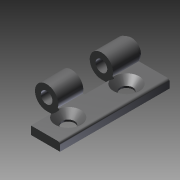
# Autodesk Inventor part: HHPMGS5p2
Saved by Autodesk Inventor 2015 SP1 (Build 190203100, 203)
## iProperties
Category: PARTsolutions
Company: MISUMI
Created: 2015-01-26
Part Number: HHPMGS5p2
Catalog Web Link: www.cadenas.de
Description: HHPMGS_p2-Low Dust Raise Hinges - Part2
Vendor: MISUMI
Document SubType Name: Modeling
Designer: PARTuser1
Manufacturer: MISUMI
Mass: 3.22136 g
Surface Area: 28.5159 cm^2
Volume: 3.22136 cm^3
Density: 1 g/cm^3
Material: Generic
Appearance: PSOLRGB-192-192-192
PSOL_IDENT_0: {\\10.0.0.236\data_v8\23d-libs\misumi\metric\39_accessories_for_al_extrusions\hhpmgs_part2.prj},167
PSOL_IDENT_1: {VTYP=3D},{NB=HHPMGS5p2},{LINA=HHPMGS5p2},{NN=HHPMGS_p2},{DATE=17.11.2014 05:31:03},{GEOMDATE=10.08.
PSOL_IDENT_2: 2009 11:07:00},{VERSION=},{LINEID=10},{LINESUBID=-1},{WBVAR=ALT1}  {NB=HHPMGS5p2},{LINA=HHPMGS5p2},{
PSOL_IDENT_3: KT=DUMMY},{PN=HHPMGS5},{TYPE=HHPMGS},{MAT=6063S-T5 Aluminum Alloy},{MATB=Oil Soaked Polyacetal},{ST=
PSOL_IDENT_4: Electroless Nickel Plating},{NO=5},{ALKG=10},{ALN=98},{MASS=22},{L=47},{W=36},{K=11.0},{P=25},{J=7.5
PSOL_IDENT_5: },{S=21},{ND=5.5},{NC=11},{T=3.5},{E=5.0},{R=5.0},{AB=FB5-8},{ABQ=4},{AN=HNTT5-5},{ANQ=4},{ALT1=},{A
PSOL_IDENT_6: BM=5},{ABL=8},{ANNO=5},{ANM=5}
SUPPLIER: MISUMI
ARTICLENO: HHPMGS5p2
BOMINFO: HHPMGS5p2
CREATOR: CADENAS GmbH
Title: HHPMGS5p2
Author: Cadenas PARTsolutions
Comments: Low Dust Raise Hinges - Part2
Autodesk Inventor part; units mm, degrees
sketch "Sketch_1" plane through (0, 0, 0) normal (0, 1, 0) x (-1, 0, 0)
  arc A0 (0, -5) -> (-4.7697, -1.5) centre (0, 0) ccw
  line L0 (-4.7697, -1.5) -> (-17, -1.5)
  arc A1 (-17, -1.5) -> (-18, -2.5) centre (-17, -2.5) ccw
  line L1 (-18, -2.5) -> (-18, -5)
  line L2 (-18, -5) -> (0, -5)
  circle A2 centre (0, 0) radius 2.5
  constraints: 6 end point, 4 point on circle, 3 centre point
extrude "Extrusion1" add sketch "Sketch_1" along normal mid plane 47
sketch "Sketch_2" plane through (0, 0, 0) normal (0, 0, 1) x (1, 0, 0)
  line L0 (-10, -23.5) -> (5.5, -23.5)
  line L1 (5.5, -23.5) -> (5.5, -11.25)
  line L2 (5.5, -11.25) -> (-5, -11.25)
  line L3 (-5, -11.25) -> (-5, -0.5)
  line L4 (-5, -0.5) -> (5.5, -0.5)
  line L5 (5.5, -0.5) -> (5.5, 12.25)
  line L6 (5.5, 12.25) -> (-5, 12.25)
  line L7 (-5, 12.25) -> (-5, 23.5)
  line L8 (-5, 23.5) -> (-10, 23.5)
  line L9 (-10, 23.5) -> (-10, -23.5)
  constraints: 20 end point
extrude "Extrusion2" cut sketch "Sketch_2" along normal mid plane 10
sketch "Sketch_4" plane through (10.5, 0, 0) normal (1, 0, 0) x (0, 0, -1)
  line L0 (5, 12.5) -> (1.5, 12.5)
  line L1 (1.5, 12.5) -> (1.5, 18)
  line L2 (1.5, 18) -> (4.25, 15.25)
  line L3 (4.25, 15.25) -> (5, 15.25)
  line L4 (5, 15.25) -> (5, 12.5)
  line L5 (5, 12.5) -> (1.5, 12.5)
  constraints: 12 end point
revolve "Revolution1" cut sketch "Sketch_4" angle 360 about axis through (10.5, 12.5, -5) along (0, 0, -1)
sketch "Sketch_5" plane through (10.5, 0, 0) normal (1, 0, 0) x (0, 0, -1)
  line L0 (5, -12.5) -> (1.5, -12.5)
  line L1 (1.5, -12.5) -> (1.5, -7)
  line L2 (1.5, -7) -> (4.25, -9.75)
  line L3 (4.25, -9.75) -> (5, -9.75)
  line L4 (5, -9.75) -> (5, -12.5)
  line L5 (5, -12.5) -> (1.5, -12.5)
  constraints: 12 end point
revolve "Revolution2" cut sketch "Sketch_5" angle 360 about axis through (10.5, -12.5, -5) along (0, 0, -1)
sketch "Sketch_10" plane through (0, 0, 0) normal (0, 0, 1) x (1, 0, 0)
  line L0 (0, 23.5) -> (0, 25.2)
  line L1 (2.5, 23.5) -> (4.5, 23.5)
  line L2 (4.5, 23.5) -> (4.5, 24.5)
  line L3 (4.5, 24.5) -> (4, 24.5)
  line L4 (4, 24.5) -> (4, 25.2)
  line L5 (4, 25.2) -> (2.5, 25.2)
  line L6 (2.5, 25.2) -> (2.5, 23.5)
  constraints: 14 end point
revolve "Revolution3" add sketch "Sketch_10" angle 360 about axis through (0, 23.5, 0) along (0, -1, 0)
ref_plane "cp_XY" through (0, 0, 0) normal (0, -1, 0) x (1, 0, 0)
ref_plane "cp_YZ" through (0, 0, 0) normal (1, 0, 0) x (0, 0, 1)
ref_plane "cp_ZX" through (0, 0, 0) normal (0, 0, 1) x (0, -1, 0)
ref_plane "bolt1_XY" through (10.5, 12.5, -4.25) normal (0, 0, 1) x (1, 0, 0)
ref_plane "bolt1_YZ" through (10.5, 12.5, -4.25) normal (1, 0, 0) x (0, 1, 0)
ref_plane "bolt1_ZX" through (10.5, 12.5, -4.25) normal (0, 1, 0) x (0, 0, 1)
ref_plane "bolt2_XY" through (10.5, -12.5, -4.25) normal (0, 0, 1) x (1, 0, 0)
ref_plane "bolt2_YZ" through (10.5, -12.5, -4.25) normal (1, 0, 0) x (0, 1, 0)
ref_plane "bolt2_ZX" through (10.5, -12.5, -4.25) normal (0, 1, 0) x (0, 0, 1)
ref_plane "nut1_XY" through (10.5, 12.5, -5) normal (0, 0, 1) x (1, 0, 0)
ref_plane "nut1_YZ" through (10.5, 12.5, -5) normal (1, 0, 0) x (0, 1, 0)
ref_plane "nut1_ZX" through (10.5, 12.5, -5) normal (0, 1, 0) x (0, 0, 1)
ref_plane "nut2_XY" through (10.5, -12.5, -5) normal (0, 0, 1) x (1, 0, 0)
ref_plane "nut2_YZ" through (10.5, -12.5, -5) normal (1, 0, 0) x (0, 1, 0)
ref_plane "nut2_ZX" through (10.5, -12.5, -5) normal (0, 1, 0) x (0, 0, 1)
body "Solid1"
